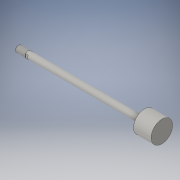
# Autodesk Inventor part: SR-094-D0_rod
Saved by Autodesk Inventor 2016 SP1 (Build 200210100, 210)
## iProperties
Category: PARTsolutions
Company: BIMBA
Created: 2017-03-15
Part Number: SR-094-D0_rod
Material: Generic
Catalog Web Link: www.cadenas.de
Description: Standard Air Cylinder_rod-Original Line - Standard Air Cylinders
Vendor: BIMBA
Document SubType Name: Standard Catalog Part
Designer: 589013
Manufacturer: BIMBA
Mass: 20.5714 g
Surface Area: 69.8864 cm^2
Volume: 20.5714 cm^3
Density: 1 g/cm^3
Appearance: PSOLRGB-181-181-181
PSOL_IDENT_0: {$CADENAS_DATA\23d-libs\bimba\bimba\bimba_imperial\bimba_full_line\original_line_cylinders\standard_
PSOL_IDENT_1: air_cylinders\rod.prj},292 {VTYP=3D},{NB=SR-094-D0_rod},{LINA=SR-094-D0_rod},{NN=Standard Air Cylind
PSOL_IDENT_2: er_rod},{DATE=09.11.2016 07:55:11},{GEOMDATE=10.09.2015 10:40:00},{VERSION=},{LINEID=10},{LINESUBID=
PSOL_IDENT_3: -1},{WBVAR=STROKE,ACTING,MNT,DER,NR,BM,CO,M,EE,EEL,K,Q,Y,F,G,T,B,H,SER,SR,NT,W,E,HL,ST,STP,PRC,PB,CO
PSOL_IDENT_4: LOR1,FCD,RCD,BCD}  {NB=SR-094-D0_rod},{LINA=SR-094-D0_rod},{KT=DUMMY},{PN=SR-094-D},{DASH=-},{BORE=1
PSOL_IDENT_5: .06250000},{BOREPN=09},{STROKE=4.000},{STROKEALG=[0.001:50/0.001]},{STROKE1=4.000},{ACTING=D},{ACTIN
PSOL_IDENT_6: GALG= '' , 'Single Acting' , 'R' , 'Reverse Single Acting' , 'D' , 'Double Acting' },{ACTINGPN=D},{M
PSOL_IDENT_7: NT=},{MNTALG= '' , 'Front Nose Mounting' , 'P' , 'Rear Pivot Mounting' , 'X' , 'Universal Pivot Moun
PSOL_IDENT_8: ting or Double End Mounting' , 'BF' , 'Front Block Mounting' , 'BR' , 'Rear Block Mounting for Verti
PSOL_IDENT_9: cal Positioning' , 'BFT' , 'Front Block Trunnion Mounting' , 'BRT' , 'Rear Block Trunnion Mounting'
PSOL_IDENT_10: },{TYPE=SR-},{MNTPN=},{DER=},{DERALG= '' , 'N/A' },{NR=},{NRALG= '' , 'N/A' },{NRPN=},{BM=},{BMALG= ''
PSOL_IDENT_11: , 'N/A' },{BMPN=},{CO=},{COALG= '' , 'N/A' },{M=},{MALG= '', 'Without Magnet', 'M', 'With Magnet' }
PSOL_IDENT_12: ,{EE=},{EEL=0},{EEMAX=46},{EEALG= '', 'Without Extra Extension', 'EE', 'With Extra Extension' },{EEL
PSOL_IDENT_13: ALG=0},{EEPN=},{EEPN1=0.000},{K=},{KALG= '', 'Standard' , 'K' , 'Ports Rotated 90deg' },{KPN=},{Q=},
PSOL_IDENT_14: {QALG= '' , 'Without Side Ported Rear Head' , 'Q' , 'With Side Ported Rear Head' },{QPN=},{Y=},{YALG=
PSOL_IDENT_15: '' , 'N/A' },{YPN=},{F=},{FALG= '', 'Standard', 'F', 'Molycoated Body' },{FPN=},{G=},{GPN=},{T=},{T
PSOL_IDENT_16: ALG= '' , 'Standard' , 'N' , 'Low Temperature' , 'V' , 'High Temperature' },{NPN=},{VPN=},{B=},{BALG=
PSOL_IDENT_17: '', 'Without Bumper' , 'B' , 'With Bumper' },{BPN=},{H=},{HALG= '', 'N/A' },{HPN=},{SER=},{SERALG= ''
PSOL_IDENT_18: , 'Without Spring Extend/Return' , 'JS' , 'With Spring Return' , 'JR' , 'With Spring Extend' },{SR=
PSOL_IDENT_19: SR},{SRALG= 'C' , 'Carbon Steel Rod' , 'SR' , '303 Stainless Steel Rod' , '' , '303 Stainless Steel
PSOL_IDENT_20: Rod1' },{SRPN=SR},{SRCON=1},{NT=},{NTPN=},{W=},{WALG= '' , 'Without Wiper' , 'W' , 'With Wiper' },{W
PSOL_IDENT_21: PN=},{E=},{EALG= '' , 'Without Special Lube and Seals' , 'E' , 'With Special Lube and Seals' },{EPN=
PSOL_IDENT_22: },{HL=},{HLALG= '' , 'Wihout Low Pressure Hydraulic' , 'HL' , 'With Low Pressure Hydraulic' },{ST=},
PSOL_IDENT_23: {STALG= '' , 'Without Switch Track' , 'T' , 'With Switch Track' },{STP=},{STPALG= '' , 'N/A' },{STPN=
PSOL_IDENT_24: },{PRC=},{PRCALG= '' , 'Without Piston Rod Clevis' , 'D-166-1' , 'With Piston Rod Clevis' },{PRCPN=}
PSOL_IDENT_25: ,{PB=},{PBALG= '' , 'Without Pivot Bracket' , 'D-167' , 'With Pivot Bracket' },{PBPN=},{TLEN=5.3125}
PSOL_IDENT_26: ,{TEXT=0.366667},{SPACE=0.209524},{FRAC=22.1200},{RGCON=},{RGDACCON=R},{RHCON=},{RHCONON=1},{RHACCON=
PSOL_IDENT_27: },{FNUTCON=1},{RNUTCON=0},{FNUTPN=D-9},{RNUTPN=},{FNUTTRANS=0.0000},{RNUTTRANS=0.0000},{VHOLECON=0},
PSOL_IDENT_28: {A1=1.6250},{A1N=1.0000},{A1P=1.6250},{A1B=1.8750},{A4=0.2525},{A4N=0.3750},{A4P=0.2525},{A5=0.0300}
PSOL_IDENT_29: ,{A1H=0.625},{A1NH=0.6250},{A1PH=1.5000},{A1BH=1.1250},{A1SH=1.1250},{A2H=0.2500},{A2NH=0.2500},{LEN
PSOL_IDENT_30: GTH=3.1200},{LENGTH1=3.1200},{LENGTH2=3.3800},{MUL=4.0000},{MUL11=4.0000},{MUL22=10.2400},{MUL33=6.2
PSOL_IDENT_31: 400},{MUL2=4.0000},{MUL211=4.0000},{MUL222=2.5600},{MUL233=1.5600},{SSS=8.0000},{RGLEN=1.4025},{RHLE
PSOL_IDENT_32: N=0.4050},{SSS1=5.0000},{A13=1.2190},{THDLEN1=0.5000},{THD1=0.3125},{TAB=UNF},{THDLEN=0.5000},{THD=0
PSOL_IDENT_33: .3125},{OD=1.0715},{RODL=7.1200},{PL=0.8700},{RODDIA=0.3120},{HEX=0.3750},{RODTRANS=0.0000},{G1=0.34
PSOL_IDENT_34: 40},{ON=0},{G5=0.7180},{DERLEN=6.1250},{THOLE=0.1900},{WF=0.2500},{BADD=0.0000},{MADD=0.0000},{NVADD=
PSOL_IDENT_35: 0.000},{JRADD=0.00000},{COLOR=0.71,0.71,0.71,0.00},{GROOVE=1},{HOL=0},{D7=0.2520},{H1=0.0000},{D1=1.
PSOL_IDENT_36: 1130},{D1RH=1.1155},{D1P=1.1410},{D1B=1.1130},{D1N=1.1130},{D1NRH=1.1155},{D1BRH=1.1410},{D1PRH=1.11
PSOL_IDENT_37: 10},{BOZO=0},{HADD=0.000},{COLOR1=0},{DEFL=0.0000},{HEXL=0.0000},{SSADD=0.1250},{WFL=0.0000},{MOVE=0
PSOL_IDENT_38: .1250},{PRCL2=0.50000},{PRCB=0.19000},{PRCTRANS=0.19000},{FCD=0},{RCD=0},{BCD=0}
NN: Standard Air Cylinder_rod
NT: Standard
NB: SR-094-D0_rod
NBSYN: $PN.$COLOR1._rod
LINA: SR-094-D0_rod
PN: SR-094-D
BORE: 1.06250000
BOREPN: 09
STROKE: 4.000
ACTING: Double Acting
MNT: Front Nose Mounting
DER: N/A
NR: N/A
BM: N/A
CO: N/A
M: Without Magnet
EE: Without Extra Extension
EEL: 0
K: Standard
Q: Without Side Ported Rear Head
Y: N/A
F: Standard
G: Without Magnalube Lubrication
T: Standard
B: Without Bumper
H: N/A
SER: Without Spring Extend/Return
SR: 303 Stainless Steel Rod
W: Without Wiper
E: Without Special Lube and Seals
HL: Wihout Low Pressure Hydraulic
ST: Without Switch Track
STP: N/A
PRC: Without Piston Rod Clevis
PB: Without Pivot Bracket
A1N: 1.0000
A1P: 1.6250
A1B: 1.8750
A4N: 0.3750
A4P: 0.2525
A5: 0.0300
A1NH: 0.6250
A1PH: 1.5000
A1BH: 1.1250
A1SH: 1.1250
A2NH: 0.2500
A13: 1.2190
THDLEN1: 0.5000
THD1: 0.3125
TAB: UNF
OD: 1.0715
RODDIA: 0.3120
HEX: 0.3750
G1: 0.3440
G5: 0.7180
THOLE: 0.1900
WF: 0.2500
GROOVE: 1
D7: 0.2520
D1P: 1.1410
D1B: 1.1130
D1N: 1.1130
D1NRH: 1.1155
D1BRH: 1.1410
D1PRH: 1.1110
COLOR1: 0
FCD: 0
RCD: 0
BCD: 0
SUPPLIER: BIMBA
ARTICLENO: SR-094-D0_rod
BOMINFO: SR-094-D0_rod
CREATOR: CADENAS GmbH
Title: SR-094-D0_rod
Author: Cadenas PARTsolutions
Comments: Original Line - Standard Air Cylinders
Autodesk Inventor part; units mm, degrees
sketch "Sketch_1" plane through (0, 0, 0) normal (0, 0, 1) x (1, 0, 0)
  line L0 (164.973, 0) -> (-3.175, 0)
  line L1 (-3.175, 0) -> (-3.175, 3.9624)
  line L2 (-3.175, 3.9624) -> (142.875, 3.9624)
  line L3 (142.875, 3.9624) -> (142.875, 13.5572)
  line L4 (142.875, 13.5572) -> (164.973, 13.5572)
  line L5 (164.973, 13.5572) -> (164.973, 0)
  line L6 (164.973, 0) -> (-3.175, 0)
  constraints: 14 end point
revolve "Revolution1" add sketch "Sketch_1" angle 360 about axis through (164.973, 0, 0) along (1, 0, 0)
sketch "Sketch_3" plane through (0, 0, 0) normal (0, 0, 1) x (1, 0, 0)
  line L0 (-3.175, 0) -> (-15.875, 0)
  line L1 (-15.875, 0) -> (-15.875, 3.3388)
  line L2 (-15.875, 3.3388) -> (-15.2451, 3.9688)
  line L3 (-15.2451, 3.9688) -> (-3.175, 3.9688)
  line L4 (-3.175, 3.9688) -> (-3.175, 0)
  line L5 (-3.175, 0) -> (-15.875, 0)
  constraints: 12 end point
revolve "Revolution2" add sketch "Sketch_3" angle 360 about axis through (-3.175, 0, 0) along (1, 0, 0)
thread "Thread1" size "5/16-24 UNF" class "2A" standard "ANSI Unified Screw Threads" full length
sketch "Sketch_10" plane through (-3.175, 0, 0) normal (1, 0, 0) x (0, 0, -1)
  line L0 (-7.9248, -7.9248) -> (7.9248, -7.9248)
  line L1 (7.9248, -7.9248) -> (7.9248, 7.9248)
  line L2 (7.9248, 7.9248) -> (-7.9248, 7.9248)
  line L3 (-7.9248, 7.9248) -> (-7.9248, -7.9248)
  line L4 (-3.175, -3.9624) -> (3.175, -3.9624)
  line L5 (3.175, -3.9624) -> (3.175, 3.9624)
  line L6 (3.175, 3.9624) -> (-3.175, 3.9624)
  line L7 (-3.175, 3.9624) -> (-3.175, -3.9624)
  constraints: 16 end point
extrude "Extrusion1" cut sketch "Sketch_10" along normal blind 3.175
ref_plane "dia1_XY" through (-3.175, 3.9624, 0) normal (1, 0, 0) x (0, 0, -1)
ref_plane "dia1_YZ" through (-3.175, 3.9624, 0) normal (0, 0, -1) x (0, 1, 0)
ref_plane "dia1_ZX" through (-3.175, 3.9624, 0) normal (0, 1, 0) x (1, 0, 0)
ref_plane "dia12_XY" through (0, 0, 14.1351) normal (1, 0, 0) x (0, 0, -1)
ref_plane "dia12_YZ" through (0, 0, 14.1351) normal (0, 0, -1) x (0, 1, 0)
ref_plane "dia12_ZX" through (0, 0, 14.1351) normal (0, 1, 0) x (1, 0, 0)
ref_plane "dia2_XY" through (-3.175, -3.9624, 0) normal (1, 0, 0) x (0, 0, -1)
ref_plane "dia2_YZ" through (-3.175, -3.9624, 0) normal (0, 0, -1) x (0, 1, 0)
ref_plane "dia2_ZX" through (-3.175, -3.9624, 0) normal (0, 1, 0) x (1, 0, 0)
ref_plane "dia22_XY" through (0, 0, -14.1351) normal (1, 0, 0) x (0, 0, -1)
ref_plane "dia22_YZ" through (0, 0, -14.1351) normal (0, 0, -1) x (0, 1, 0)
ref_plane "dia22_ZX" through (0, 0, -14.1351) normal (0, 1, 0) x (1, 0, 0)
ref_plane "rl1_XY" through (-15.875, 0, 0) normal (1, 0, 0) x (0, 0, -1)
ref_plane "rl1_YZ" through (-15.875, 0, 0) normal (0, 0, -1) x (0, 1, 0)
ref_plane "rl1_ZX" through (-15.875, 0, 0) normal (0, 1, 0) x (1, 0, 0)
ref_plane "rl2_XY" through (-3.175, 0, 0) normal (1, 0, 0) x (0, 0, -1)
ref_plane "rl2_YZ" through (-3.175, 0, 0) normal (0, 0, -1) x (0, 1, 0)
ref_plane "rl2_ZX" through (-3.175, 0, 0) normal (0, 1, 0) x (1, 0, 0)
ref_plane "rod_cp_XY" through (0, 0, 0) normal (1, 0, 0) x (0, 0, -1)
ref_plane "rod_cp_YZ" through (0, 0, 0) normal (0, 0, -1) x (0, 1, 0)
ref_plane "rod_cp_ZX" through (0, 0, 0) normal (0, 1, 0) x (1, 0, 0)
ref_plane "thd1_XY" through (-15.875, 3.9688, 0) normal (1, 0, 0) x (0, 0, -1)
ref_plane "thd1_YZ" through (-15.875, 3.9688, 0) normal (0, 0, -1) x (0, 1, 0)
ref_plane "thd1_ZX" through (-15.875, 3.9688, 0) normal (0, 1, 0) x (1, 0, 0)
ref_plane "thd2_XY" through (-15.875, -3.9688, 0) normal (1, 0, 0) x (0, 0, -1)
ref_plane "thd2_YZ" through (-15.875, -3.9688, 0) normal (0, 0, -1) x (0, 1, 0)
ref_plane "thd2_ZX" through (-15.875, -3.9688, 0) normal (0, 1, 0) x (1, 0, 0)
ref_plane "to_rod_clevis_XY" through (-20.701, 0, 0) normal (1, 0, 0) x (0, 0, -1)
ref_plane "to_rod_clevis_YZ" through (-20.701, 0, 0) normal (0, 0, -1) x (0, 1, 0)
ref_plane "to_rod_clevis_ZX" through (-20.701, 0, 0) normal (0, 1, 0) x (1, 0, 0)
ref_plane "wf1_XY" through (-3.175, 0, 0) normal (1, 0, 0) x (0, 0, -1)
ref_plane "wf1_YZ" through (-3.175, 0, 0) normal (0, 0, -1) x (0, 1, 0)
ref_plane "wf1_ZX" through (-3.175, 0, 0) normal (0, 1, 0) x (1, 0, 0)
ref_plane "wf2_XY" through (0, 0, 0) normal (1, 0, 0) x (0, 0, -1)
ref_plane "wf2_YZ" through (0, 0, 0) normal (0, 0, -1) x (0, 1, 0)
ref_plane "wf2_ZX" through (0, 0, 0) normal (0, 1, 0) x (1, 0, 0)
ref_plane "wfw1_XY" through (-3.175, 0, -3.175) normal (0, 1, 0) x (1, 0, 0)
ref_plane "wfw1_YZ" through (-3.175, 0, -3.175) normal (1, 0, 0) x (0, 0, -1)
ref_plane "wfw1_ZX" through (-3.175, 0, -3.175) normal (0, 0, -1) x (0, 1, 0)
ref_plane "wfw2_XY" through (-3.175, 0, 3.175) normal (0, 1, 0) x (1, 0, 0)
ref_plane "wfw2_YZ" through (-3.175, 0, 3.175) normal (1, 0, 0) x (0, 0, -1)
ref_plane "wfw2_ZX" through (-3.175, 0, 3.175) normal (0, 0, -1) x (0, 1, 0)
body "Solid1"
